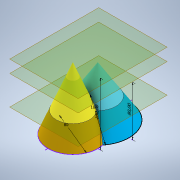
# Autodesk Inventor part: Деталь2
Saved by Autodesk Inventor 2021.2 (Build 252289000, 289)
## iProperties
Created: 2023-11-20
Part Number: Деталь2
Material: Типовые
Document SubType Name: Modeling
Designer: pekav
Density: 1 g/cm^3
Appearance: По умолчанию
Author: pekav
Autodesk Inventor part; units mm, degrees
ref_plane "YZ Plane" through (0, 0, 0) normal (1, 0, 0) x (0, 1, 0)
ref_plane "XZ Plane" through (0, 0, 0) normal (0, 1, 0) x (-1, 0, 0)
ref_plane "XY Plane" through (0, 0, 0) normal (0, 0, 1) x (1, 0, 0)
sketch "Эскиз1" plane through (0, 0, 0) normal (0, 1, 0) x (-1, 0, 0)
  circle A0 centre (0, 0) radius 50
  circle A1 centre (0, 40) radius 40
  line L0 (44.1832, 40) -> (-44.0888, 40)
  line L1 (0.3076, 84.5902) -> (0.3076, -55.7597)
  line L2 (55.3799, 0) -> (-56.0667, 0)
  dimension "d0" = 100
  dimension "d2" = 80
  constraints: 6 end point, 2 centre point, 2 horizontal, 1 coincident, 1 vertical
  measures "d0" diameter of A0
  measures "d2" diameter of A1
sketch "Эскиз2" plane through (0, 0, 0) normal (1, 0, 0) x (0, 1, 0)
  line L0 (0, 40.0046) -> (100, 40.0046)
  line L1 (0, 40.0046) -> (0, 80.0046)
  line L2 (0, 80.0046) -> (100, 40.0046)
  line L3 (0, 0) -> (80, 0)
  line L4 (0, 0) -> (0, -50)
  line L5 (0, -50) -> (80, 0)
  dimension "d3" = 100
  dimension "d4" = 40
  dimension "d5" = 80
  dimension "d6" = 50
  constraints: 12 end point, 2 horizontal, 2 vertical
  measures "d3" distance of L0.start L0.end
  measures "d4" distance of L0.start L1.end
  measures "d5" distance of L3.start L3.end
  measures "d6" distance of L3.start L4.end
revolve "Вращение1" add sketch "Эскиз2" angle 360 about axis through (0, 0, 40.0046) along (0, 1, 0) contours L1 L2 L0
revolve "Вращение2" add sketch "Эскиз2" angle 360 about axis through (0, 0, 0) along (0, 1, 0) contours L3 L5 L4
ref_plane "РабПлоскость1" through (0, 33.25, 0) normal (0, -1, 0) x (1, 0, 0)
split_face "Разделение1"
split_face "Разделение2"
ref_plane "РабПлоскость2" through (0, 100, 0) normal (0, -1, 0) x (1, 0, 0)
ref_plane "РабПлоскость3" through (0, 80, 0) normal (0, -1, 0) x (1, 0, 0)
